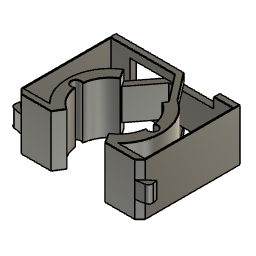
omega clamp (Autodesk Fusion 360 design; units mm, degrees)
Autodesk Fusion 360 part; units mm, degrees
note: some values were not read from the file. Set by a fixed rule: which sketch regions a step uses.
sketch "Sketch1" plane through (0, 0, 0) normal (0, 0, 1) x (1, 0, 0)
  arc A0 (-7.893051, 12.755381) -> (-14.903374, 1.699834) centre (0, 0) ccw
  arc A1 (-14.903374, 1.699834) -> (-14.903374, -1.699834) centre (-16.3, 0) ccw
  arc A2 (-14.903374, -1.699834) -> (-7.893051, -12.755381) centre (0, 0) ccw
  line L0 (0, 0) -> (-44.000001, 0) construction
  arc A3 (-10.78717, 17.432354) -> (-10.78717, -17.432354) centre (0, 0) ccw
  line L1 (-7.893051, -12.755381) -> (-10.78717, -17.432354)
  line L2 (-7.893051, 12.755381) -> (-10.78717, 17.432354)
  line L3 (0, 0) -> (-7.893051, -12.755381) construction
  line L4 (0, 0) -> (-7.893051, 12.755381) construction
  point P0 (-18.5, 0)
  point P1 (-14.5, 0)
  point P2 (-20.5, 0)
  dimension "d12" = 2.2
  dimension "d14" = 4
  dimension "d15" = 2
  dimension "d80" = 30
  dimension "d82" = 3.399668
  dimension "d83" = 116.50142
  constraint coincident A0.centre A2.centre
  constraint horizontal L0
  constraint coincident A1.centre L0
  constraint midpoint A1 P0
  constraint coincident L0 P1
  constraint coincident L0 P2
  constraint coincident A3 P2
  constraint midpoint A3 P2
  constraint coincident A0.centre L1
  constraint parallel L2 L4
  constraint equal A0 A2
  measures "d12" radius of A1
  measures "d14" distance of P0 P1
  measures "d15" distance of P0 P2
  measures "d80" diameter of A0
  measures "d83" angle of L3 L4
extrude "Extrude1" add sketch "Sketch1" along normal blind 25 makes body 1
ref_plane "WorkPlane1" through (-14.903374, 1.699834, 12.5) normal (-1, 0, 0) x (0, 0, 1)
ref_plane "WorkPlane2" through (2.096626, 1.699834, 12.5) normal (-1, 0, 0) x (0, 0, 1)
mirror "Mirror1" about plane through (2.096626, 1.699834, 12.5) normal (-1, 0, 0) of bodies 1 makes body 2
sketch "Sketch2" plane through (0, 0, 0) normal (0, 0, 1) x (1, 0, 0)
  arc A0 (-10.78717, 17.432354) -> (-10.78717, -17.432354) centre (0, 0) ccw
  arc A1 (-14.903374, -1.699834) -> (-7.893051, -12.755381) centre (0, 0) ccw
  arc A2 (-14.903374, 1.699834) -> (-14.903374, -1.699834) centre (-16.3, 0) ccw
  arc A3 (-7.893051, 12.755381) -> (-14.903374, 1.699834) centre (0, 0) ccw
  arc A4 (19.096626, 1.699834) -> (12.086303, 12.755381) centre (4.193252, 0) ccw
  arc A5 (19.096626, -1.699834) -> (19.096626, 1.699834) centre (20.493252, 0) ccw
  arc A6 (12.086303, -12.755381) -> (19.096626, -1.699834) centre (4.193252, 0) ccw
  arc A7 (14.980421, -17.432354) -> (14.980421, 17.432354) centre (4.193252, 0) ccw
  line L0 (-10.78717, -17.432354) -> (-27.558748, -17.432354)
  line L1 (-27.558748, -17.432354) -> (-27.558748, -14.432354)
  line L2 (-27.558748, -14.432354) -> (-14.558748, -14.432354)
  line L3 (-27.558748, -14.432354) -> (-27.558748, 27.432354)
  line L4 (-26.958748, 27.432354) -> (-26.958748, -14.432354)
  line L5 (-27.558748, 27.432354) -> (3.503217, 27.432354)
  line L6 (-27.558748, 27.432354) -> (-27.558748, 30.432354)
  line L7 (-27.558748, 30.432354) -> (4.980421, 30.432354)
  line L8 (4.980421, 30.432354) -> (14.980421, 17.432354)
  line L9 (3.503217, 27.432354) -> (13.293068, 14.705547)
  line L10 (-10.78717, -17.432354) -> (-6.962502, -17.432354)
  line L11 (-25.058748, -17.432354) -> (-27.558748, -14.932354)
  line L12 (-6.962502, -17.432354) -> (36.000001, -17.432354)
  line L13 (-7.893051, 12.755381) -> (-10.78717, 17.432354)
  line L14 (-10.78717, -17.432354) -> (-7.893051, -12.755381)
  line L15 (12.086303, -12.755381) -> (14.980421, -17.432354)
  line L16 (14.980421, 17.432354) -> (12.086303, 12.755381)
  dimension "d40" = 3
  dimension "d41" = 0.6
  dimension "d42" = 3
  dimension "d43" = 3
  dimension "d45" = 10
  dimension "d46" = 10
  dimension "d47" = 41.864708
  dimension "d48" = 13
  dimension "d49" = 45
  dimension "d50" = 0.5
  constraint horizontal L0
  constraint perpendicular L0 L1
  constraint perpendicular L1 L2
  constraint perpendicular L2 L3
  constraint perpendicular L2 L4
  constraint perpendicular L4 L5
  constraint perpendicular L5 L6
  constraint perpendicular L6 L7
  constraint parallel L8 L9
  constraint horizontal L10
  constraint parallel L10 L12
  measures "d41" distance of L3 L4
  measures "d42" distance of L8 L9
  measures "d43" distance of L5 L7
  measures "d49" angle of L0 L11
extrude "Extrude2" add sketch "Sketch2" along normal up to surface (25 mm away) separate body contours A0 L0 L1 L2 L11 | L2 L3 L4 L5 | L5 L6 L7 L8 L9 L16 picked at (-22.192082, -15.432354) picked at (-27.158748, -0.477451) picked at (-6.35837, 29.432354) makes body 3
ref_plane "WorkPlane3" through (-6.289164, 6.5, 12.5) normal (0, 0, 1) x (1, 0, 0)
sketch "Sketch4" plane through (-6.489814, 5.500004, 12.5) normal (0, 0, 1) x (1, 0, 0)
  line L0 (21.470235, 11.93235) -> (11.470235, 24.93235)
  line L1 (11.470235, 24.93235) -> (-21.068935, 24.93235)
  line L2 (-21.068935, 24.93235) -> (-21.068935, -20.432359)
  line L3 (-21.068935, -20.432359) -> (-18.568935, -22.932359)
  line L4 (-18.568935, -22.932359) -> (-4.297356, -22.932359)
  arc A0 (-8.068935, -19.932359) -> (-4.297356, -22.932359) centre (6.489814, -5.500004) ccw
  line L5 (-18.568935, -22.932359) -> (-22.791483, -22.187809)
  line L6 (-24.413802, -19.870898) -> (-24.068935, -17.91506)
  line L7 (-24.068935, -17.91506) -> (-21.068935, -20.432359)
  arc A1 (-24.413802, -19.870898) -> (-22.791483, -22.187809) centre (-22.444186, -20.218194) ccw
  line L8 (19.782882, 9.205543) -> (21.470235, 11.93235)
  line L9 (-8.068935, -19.932359) -> (-20.468935, -19.932359)
  line L10 (-20.468935, -19.932359) -> (-20.468935, 21.93235)
  line L11 (-20.468935, 21.93235) -> (9.99303, 21.93235)
  line L12 (9.99303, 21.93235) -> (19.782882, 9.205543)
  dimension "d69" = 2
  dimension "d70" = 3
  dimension "d72" = 50
  dimension "d73" = 10
  constraint perpendicular L5 L6
  constraint tangent L5 A1
  constraint tangent L6 A1
  measures "d69" radius of A1
  measures "d72" angle of L2 L7
  measures "d73" angle of L4 L5
extrude "Extrude7" add sketch "Sketch4" along normal mid plane 8 contours L3 L5 L6 L7 A1 picked at (-20.809784, -21.850842) bodies 3
mirror "Mirror2" about plane through (2.096626, 1.699834, 12.5) normal (-1, 0, 0) of bodies 3 makes body 4
sketch "Sketch3" plane through (0, 30.432354, 0) normal (0, 1, 0) x (-1, 0, 0)
  line L0 (0.78717, 25) -> (-31.752, 25)
  line L1 (-31.752, 0) -> (0.78717, 0)
  line L2 (27.558748, 25) -> (-4.980421, 25)
  line L3 (-4.980421, 0) -> (27.558748, 0)
  line L4 (27.558748, 4) -> (-31.752, 4)
  line L5 (27.558748, 5) -> (-31.752, 5)
  line L6 (-31.752, 20) -> (27.558748, 20)
  line L7 (27.558748, 21) -> (-31.752, 21)
  line L8 (-2.096626, 4) -> (-2.096626, 5) construction
  line L9 (-2.096626, 20) -> (-2.096626, 21) construction
  line L10 (-2.096626, 21) -> (-2.096626, 25) construction
  line L11 (-2.096626, 4) -> (-2.096626, 0) construction
  line L12 (10.78717, 25) -> (0.78717, 25)
  line L13 (0.78717, 0) -> (10.78717, 0)
  line L14 (27.558748, 0) -> (27.558748, 25)
  line L15 (17.903374, 25) -> (17.903374, 0)
  line L16 (-22.096626, 0) -> (-22.096626, 25)
  line L17 (-22.096626, 0) -> (17.903374, 0) construction
  line L18 (10.78717, 0) -> (10.78717, 25)
  line L19 (-31.752, 0) -> (-31.752, 25)
  dimension "d58" = 1
  dimension "d59" = 4
  dimension "d78" = 40
  constraint perpendicular L7 L10
  constraint perpendicular L4 L11
  constraint equal L10 L11
  constraint equal L8 L9
  constraint perpendicular L7 L14
  constraint horizontal L6
  constraint perpendicular L5 L14
  constraint vertical L8
  constraint perpendicular L3 L15
  constraint perpendicular L0 L16
  constraint perpendicular L15 L17
  constraint coincident L1.start L19.start
  constraint coincident L0.end L19.end
  constraint coincident L5.end L19
  constraint coincident L6.start L19
  constraint coincident L7.end L19
  measures "d58" distance of L4 L5
extrude "Extrude5" cut sketch "Sketch3" against normal blind 20 contours L0 L2 L7 L12 L16 L18 | L2 L7 L15 L18 | L6 L7 L16 L18 | L6 L7 L15 L18 | L4 L5 L16 L18 | L4 L5 L15 L18 | L1 L3 L4 L13 L16 L18 | L3 L4 L15 L18 picked at (-5.429959, 22.333333) picked at (13.159238, 23.666667) picked at (-0.174095, 20.666667) picked at (15.531306, 20.333333) picked at (-0.174095, 4.666667) picked at (15.531306, 4.666667) picked at (-3.507429, 2.666667) picked at (15.531306, 1.333333) bodies 4
extrude "Extrude6" cut sketch "Sketch3" against normal blind 25 contours L6 L7 L16 L18 | L6 L7 L15 L18 | L5 L6 L16 L18 | L5 L6 L15 L18 | L4 L5 L16 L18 | L4 L5 L15 L18 picked at (-0.174095, 20.666667) picked at (15.531306, 20.333333) picked at (-11.135361, 10) picked at (13.159238, 10) picked at (-0.174095, 4.666667) picked at (15.531306, 4.666667) bodies 3
combine "Combine1" operation add target body 1 tool bodies 2 3 4
chamfer "Chamfer3" distance 0.2 angle 45 2 faces at (-11.604812, -14.499529, 0) (-11.604812, -14.499529, 25) on bodies 1
equation "rubber_width = 29.5 mm"
equation "shaft_diameter = 30 mm"
equation "chord_angle = ( ( rubber_width + slop ) / ( shaft_diameter * PI ) * 2 * PI ) * 1 rad"
equation "d80 = shaft_diameter"
equation "slop = 1 mm"
equation "d83 = chord_angle"
named bodies: "omega clamp"
